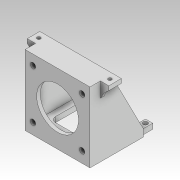
# Autodesk Inventor part: J2MotorBracket_56mm
Saved by Autodesk Inventor 2020 (Build 240168000, 168)
## iProperties
Created: 2021-11-21
Part Number: J2MotorBracket_56mm
Material: Generic
Document SubType Name: Modeling
Designer: DDeGo
Density: 1 g/cm^3
Appearance: Default
Author: DDeGo
Autodesk Inventor part; units mm, degrees
ref_plane "YZ Plane" through (0, 0, 0) normal (1, 0, 0) x (0, 1, 0)
ref_plane "XZ Plane" through (0, 0, 0) normal (0, 1, 0) x (-1, 0, 0)
sketch "Sketch1" plane through (0, 0, 0) normal (0, 0, 1) x (1, 0, 0)
  line L0 (-23.5, -23.5) -> (23.5, -23.5) construction
  line L1 (23.5, -23.5) -> (23.5, 23.5) construction
  line L2 (23.5, 23.5) -> (-23.5, 23.5) construction
  line L3 (-23.5, 23.5) -> (-23.5, -23.5) construction
  line L4 (-23.5, -23.5) -> (23.5, 23.5) construction
  line L5 (23.5, -23.5) -> (-23.5, 23.5) construction
  circle A0 centre (0, 0) radius 20
  circle A1 centre (-23.5, 23.5) radius 2.6
  circle A2 centre (23.5, 23.5) radius 2.6
  circle A3 centre (23.5, -23.5) radius 2.6
  circle A4 centre (-23.5, -23.5) radius 2.6
  line L6 (29, 29) -> (-29, 29)
  line L7 (-29, 29) -> (-29, -29)
  line L8 (-29, -29) -> (29, -29)
  line L9 (29, -29) -> (29, 29)
  line L10 (29, 29) -> (-29, -29) construction
  line L11 (-29, 29) -> (29, -29) construction
  dimension "d0" = 5.2
  dimension "d1" = 47
  dimension "d2" = 47
  dimension "d3" = 40
  dimension "d4" = 58
  constraints: 24 end point, 5 centre point, 5 coincident, 4 midpoint, 4 parallel, 3 equal radius, 2 horizontal, 2 perpendicular, 1 point on line
  measures "d0" diameter of A1
  measures "d1" distance of L1.end L2.end
  measures "d2" distance of L0.end L1.end
  measures "d3" diameter of A0
  measures "d4" distance of L6.start L6.end
extrude "Extrusion1" add sketch "Sketch1" along normal blind 3.5
sketch "Sketch2" plane through (-29, 29, 0) normal (0, 1, 0) x (1, 0, 0)
  line L0 (58, 0) -> (0, 0) construction
  line L1 (0, 0) -> (0, -3.5) construction
  line L2 (58, -3.5) -> (0, -3.5) projected
  line L3 (58, 0) -> (58, -3.5) construction
  line L4 (58, -3.5) -> (0, -3.5) projected
  line L5 (0, -3.5) -> (-10, -3.5)
  line L6 (-10, -3.5) -> (-10, 8.5)
  line L7 (-10, 8.5) -> (68, 8.5)
  line L8 (68, 8.5) -> (68, -3.5)
  line L9 (68, -3.5) -> (58, -3.5)
  point P0 (29, 0)
  dimension "d7" = 10
  dimension "d8" = 12
  constraints: 10 end point, 4 perpendicular, 1 collinear, 1 horizontal, 1 point on line
  measures "d7" distance of L1.end L5.end
  measures "d8" distance of L5.end L6.end
extrude "Extrusion2" add sketch "Sketch2" along normal blind 4
sketch "Sketch3" plane through (-39, 29, -8.5) normal (-1, 0, 0) x (0, 0, 1)
  line L0 (0, 0) -> (12, 0) projected
  line L1 (12, 0) -> (12, -58) construction
  line L2 (12, 0) -> (12, -8.5)
  line L3 (12, -8.5) -> (8.5, -8.5)
  line L4 (8.5, -8.5) -> (0, 0)
  line L5 (8.5, 0) -> (12, 0) projected
  point P0 (8.5, -29)
  dimension "d20" = 45
  constraints: 6 end point, 1 horizontal, 1 parallel, 1 point on line, 1 vertical
  measures "d20" angle of L0 L4
extrude "Extrusion3" add sketch "Sketch3" against normal up to surface (10 mm away)
sketch "Sketch4" plane through (0, 0, 3.5) normal (0, 0, 1) x (1, 0, 0)
  line L0 (-29, 20.5) -> (-39, 29)
  line L1 (-39, 20.5) -> (-39, 33) construction
  line L2 (-39, 29) -> (-39, 20.5)
  line L3 (-39, 20.5) -> (-29, 20.5) projected
  point P0 (0, 0)
  constraints: 4 end point, 1 coincident, 1 point on line, 1 vertical
extrude "Extrusion4" cut sketch "Sketch4" against normal through all
mirror "Mirror1" about plane through (0, 0, 0) normal (1, 0, 0) of "Extrusion3", "Extrusion4"
fillet "Fillet1" radius 25 2 edges at (-29, 20.5, 1.75) (29, 20.5, 1.75)
sketch "Sketch5" plane through (-29, 33, 0) normal (0, 1, 0) x (1, 0, 0)
  line L0 (68, -3.5) -> (68, 8.5) construction
  line L1 (68, 2.5) -> (-10, 2.5) construction
  line L2 (-10, 8.5) -> (-10, -3.5) construction
  circle A0 centre (63, 2.5) radius 1.65
  circle A1 centre (-5, 2.5) radius 1.65
  point P0 (29, 0)
  dimension "d22" = 5
  dimension "d23" = 5
  dimension "d24" = 3.3
  constraints: 2 centre point, 2 end point, 2 midpoint, 2 point on line, 1 equal radius
  measures "d22" distance from line of L2 A1.centre
  measures "d23" distance from line of A0.centre L0
  measures "d24" diameter of A1
extrude "Extrusion5" cut sketch "Sketch5" against normal through all
ref_plane "Work Plane1" through (-29, 26.5, 0) normal (0, 1, 0) x (1, 0, 0)
sketch "Sketch6" plane through (-29, 26.5, 0) normal (0, -1, 0) x (1, 0, 0)
  circle A0 centre (63, -2.5) radius 1.65 projected
  circle A1 centre (-5, -2.5) radius 1.65 projected
  circle A2 centre (63, -2.5) radius 3
  arc A3 (-5.4929, -4.0747) -> (-3.6851, -1.5032) centre (-5, -2.5) ccw projected
  circle A4 centre (-5, -2.5) radius 3
  point P0 (29, 0)
  dimension "d27" = 6
  constraints: 2 centre point, 2 coincident, 1 equal radius
  measures "d27" diameter of A2
extrude "Extrusion6" cut sketch "Sketch6" along normal blind 10 contours A0 | A1 | A2 | A4
sketch "Sketch7" plane through (-29, -29, 0) normal (0, -1, 0) x (1, 0, 0)
  line L0 (0, 3.5) -> (58, 3.5) projected
  line L1 (0, 3.5) -> (58, 3.5)
  line L2 (58, 3.5) -> (58, -47.5)
  line L3 (51, -41.3) -> (7, -41.3)
  line L4 (0, -47.5) -> (0, 3.5)
  line L5 (29, -41.3) -> (29, 3.5) construction
  line L6 (11, -35.3) -> (47, -35.3)
  line L7 (52, -30.3) -> (52, -7.5)
  line L8 (47, -2.5) -> (11, -2.5)
  line L9 (6, -7.5) -> (6, -30.3)
  line L10 (6, -35.3) -> (52, -2.5) construction
  line L11 (52, -35.3) -> (6, -2.5) construction
  line L12 (0, 0) -> (58, 0) construction
  circle A0 centre (63, -2.5) radius 1.65 construction
  line L13 (0, -47.5) -> (0, -48.5)
  line L14 (0, -48.5) -> (7, -48.5)
  line L15 (7, -48.5) -> (7, -41.3)
  line L16 (58, -47.5) -> (58, -48.5)
  line L17 (58, -48.5) -> (51, -48.5)
  line L18 (51, -48.5) -> (51, -41.3)
  arc A1 (11, -2.5) -> (6, -7.5) centre (11, -7.5) ccw
  arc A2 (6, -30.3) -> (11, -35.3) centre (11, -30.3) ccw
  arc A3 (47, -35.3) -> (52, -30.3) centre (47, -30.3) ccw
  arc A4 (52, -7.5) -> (47, -2.5) centre (47, -7.5) ccw
  point P0 (29, 0)
  point P1 (29, -18.9)
  dimension "d32" = 6
  dimension "d33" = 6
  dimension "d35" = 7.2
  dimension "d36" = 7
  dimension "d39" = 44.8
  dimension "d40" = 5
  dimension "d41" = 6
  constraints: 34 end point, 8 point on circle, 8 point on line, 8 tangent, 6 midpoint, 6 perpendicular, 4 centre point, 4 parallel, 3 equal radius, 2 equal length, 2 horizontal, 2 vertical
  measures "d32" distance between parallel lines of L2 L7
  measures "d33" distance between parallel lines of L3 L6
  measures "d35" distance between parallel lines of L3 L17
  measures "d36" distance of L16.end L17.end
  measures "d39" distance between parallel lines of L3 L0
  measures "d40" radius of A1
  measures "d41" distance between parallel lines of L0 L8
extrude "Extrusion7" add sketch "Sketch7" along normal blind 5
sketch "Sketch8" plane through (-29, -34, 0) normal (0, -1, 0) x (1, 0, 0)
  line L0 (0, -48.5) -> (7, -48.5) construction
  line L1 (3.5, -48.5) -> (3.5, -45) construction
  line L2 (51, -48.5) -> (58, -48.5) construction
  line L3 (54.5, -48.5) -> (54.5, -45) construction
  circle A0 centre (3.5, -45) radius 2.15
  circle A1 centre (54.5, -45) radius 2.15
  point P0 (29, 0)
  dimension "d42" = 3.5
  dimension "d43" = 4.3
  constraints: 4 end point, 2 centre point, 2 coincident, 2 midpoint, 2 vertical, 1 equal radius, 1 parallel
  measures "d42" distance of L1.start L1.end
  measures "d43" diameter of A0
extrude "Extrusion8" cut sketch "Sketch8" against normal blind 5
sketch "Sketch9" plane through (-29, 8.939, 0) normal (-1, 0, 0) x (0, 0, 1)
  line L0 (0, 11.061) -> (0, -28.939) construction
  line L1 (-8.5, 20.061) -> (3.5, 20.061)
  line L2 (3.5, 0) -> (3.5, -42.939) projected
  line L3 (3.5, -42.939) -> (-48.5, -42.939) construction
  line L4 (3.5, 20.061) -> (3.5, -42.939)
  line L5 (3.5, -42.939) -> (-38.5, -42.939)
  line L6 (-38.5, -42.939) -> (-38.5, -37.939)
  line L7 (0, -37.939) -> (-48.5, -37.939) construction
  line L8 (-8.5, 20.061) -> (-38.5, -37.939)
  point P0 (0, -8.939)
  dimension "d56" = 42
  constraints: 10 end point, 2 perpendicular, 2 point on line, 1 coincident, 1 horizontal, 1 vertical
  measures "d56" distance between parallel lines of L2 L6
extrude "Extrusion9" add sketch "Sketch9" along normal blind 2
chamfer "Chamfer2" distance 1 angle 45 1 edges at (-31, -31.5, -38.5)
mirror "Mirror2" about plane through (0, 0, 0) normal (1, 0, 0) of "Extrusion9", "Chamfer2"
sketch "Sketch10" plane through (0, 0, 3.5) normal (0, 0, 1) x (1, 0, 0)
  circle A0 centre (-23.5, -23.5) radius 2.6 projected
  circle A1 centre (23.5, -23.5) radius 2.6 projected
  circle A2 centre (23.5, 23.5) radius 2.6 projected
  circle A3 centre (-23.5, 23.5) radius 2.6 projected
  circle A4 centre (0, 0) radius 20 projected
  arc A5 (37.8088, 27.9875) -> (31, 18.7369) centre (54, 8.939) ccw construction
  line L0 (37.8088, 27.9875) -> (39, 29) construction
  line L1 (39, 29) -> (39, 33) construction
  line L2 (-39, 33) -> (39, 33) projected
  line L3 (-39, 29) -> (-39, 33) construction
  line L4 (-39, 29) -> (-37.8088, 27.9875) construction
  arc A6 (-31, 18.7369) -> (-37.8088, 27.9875) centre (-54, 8.939) ccw construction
  line L5 (-31, -34) -> (-31, 18.7369) projected
  line L6 (-31, -34) -> (31, -34) projected
  line L7 (31, -34) -> (31, 18.7369) projected
  arc A7 (31.8337, 20.5) -> (31, 18.7369) centre (54, 8.939) ccw projected
  line L8 (31, 18.7369) -> (31, 33)
  line L9 (-31, -34) -> (-31, 18.7369) projected
  line L10 (-31, 18.7369) -> (-31, 33)
  line L11 (39, 33) -> (-39, 33) projected
  constraints: 4 end point, 2 point on line, 1 parallel, 1 perpendicular
extrude "Extrusion10" add sketch "Sketch10" along normal blind 10
sketch "Sketch11" plane through (0, 0, 0) normal (0, 0, -1) x (-1, 0, 0)
  line L0 (-29, -29) -> (-29, 29) projected
  line L1 (29, -29) -> (-29, -29) projected
  line L2 (29, 29) -> (29, -29) projected
  line L3 (-29, 29) -> (29, 29) projected
  circle A0 centre (23.5, -23.5) radius 2.6 projected
  circle A1 centre (-23.5, -23.5) radius 2.6 projected
  circle A2 centre (-23.5, 23.5) radius 2.6 projected
  circle A3 centre (23.5, 23.5) radius 2.6 projected
  circle A4 centre (0, 0) radius 20 projected
extrude "Extrusion11" cut sketch "Sketch11" against normal blind 10 contours L0 L3 L2 L1 | A0 | A1 | A2 | A3 | A4
equation "\"d23\" = d22"
equation "\"d32\" = d41"
equation "\"d33\" = d41"
body "Solid1"
